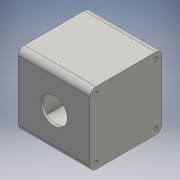
# Autodesk Inventor part: 60x60Motor
Saved by Autodesk Inventor 2016 (Build 200138000, 138)
## iProperties
Created: 2016-05-22
Part Number: 60x60Motor
Material: Generic
Document SubType Name: Modeling
Designer: Kurtis
Density: 1 g/cm^3
Appearance: Default
Author: Kurtis
Autodesk Inventor part; units mm, degrees
ref_plane "YZ Plane" through (0, 0, 0) normal (1, 0, 0) x (0, 1, 0)
ref_plane "XZ Plane" through (0, 0, 0) normal (0, 1, 0) x (-1, 0, 0)
ref_plane "XY Plane" through (0, 0, 0) normal (0, 0, 1) x (1, 0, 0)
sketch "Sketch1" plane through (0, 0, 0) normal (0, 0, 1) x (1, 0, 0)
  line L0 (-30, -30) -> (30, -30)
  line L1 (30, -30) -> (30, 30)
  line L2 (30, 30) -> (-30, 30)
  line L3 (-30, 30) -> (-30, -30)
  line L4 (-30, -30) -> (30, 30) construction
  line L5 (30, -30) -> (-30, 30) construction
  point P0 (0, 0)
  dimension "d0" = 60
  dimension "d1" = 60
  constraints: 12 end point, 2 midpoint, 2 parallel, 1 horizontal, 1 perpendicular
  measures "d0" distance of L2.end L1.end
  measures "d1" distance of L1.end L0.end
extrude "Main Block" add sketch "Sketch1" along normal blind 60
sketch "Sketch2" plane through (-30, 30, 0) normal (0, 1, 0) x (1, 0, 0)
  line L0 (0, -60) -> (60, -60) construction
  line L1 (0, 0) -> (60, 0) construction
  line L2 (60, -60) -> (0, 0) construction
  line L3 (51.25, -51.25) -> (8.75, -51.25)
  line L4 (8.75, -51.25) -> (8.75, -8.75)
  line L5 (8.75, -8.75) -> (51.25, -8.75)
  line L6 (51.25, -8.75) -> (51.25, -51.25)
  line L7 (51.25, -51.25) -> (8.75, -8.75) construction
  line L8 (8.75, -51.25) -> (51.25, -8.75) construction
  line L9 (30, -30) -> (30, -51.25) construction
  point P0 (30, 0)
  dimension "d4" = 42.5
  dimension "d5" = 42.5
  constraints: 16 end point, 4 midpoint, 2 parallel, 1 horizontal, 1 perpendicular
  measures "d4" distance of L4.end L5.end
  measures "d5" distance of L3.end L4.end
extrude "Motor Void" cut sketch "Sketch2" against normal blind 58
sketch "Sketch3" plane through (-30, 30, 0) normal (0, 1, 0) x (1, 0, 0)
  line L0 (30, 0) -> (30, -8.75) construction
  line L1 (8.75, -8.75) -> (51.25, -8.75) construction
  line L2 (38.25, 0.125) -> (21.75, 0.125)
  line L3 (21.75, 0.125) -> (21.75, -8.875)
  line L4 (21.75, -8.875) -> (38.25, -8.875)
  line L5 (38.25, -8.875) -> (38.25, 0.125)
  line L6 (38.25, 0.125) -> (21.75, -8.875) construction
  line L7 (21.75, 0.125) -> (38.25, -8.875) construction
  point P0 (30, -4.375)
  dimension "d30" = 16.5
  dimension "d31" = 9
  constraints: 14 end point, 4 midpoint, 2 parallel, 1 horizontal, 1 perpendicular
  measures "d30" distance of L4.end L3.end
  measures "d31" distance of L3.end L2.end
extrude "Cable Void" cut sketch "Sketch3" against normal blind 41
sketch "Sketch4" plane through (-30, -30, 0) normal (0, -1, 0) x (1, 0, 0)
  line L0 (0, 0) -> (0, 60) construction
  line L1 (60, 60) -> (0, 60) construction
  line L2 (0, 0) -> (60, 60) construction
  circle A0 centre (30, 30) radius 11
  point P0 (30, 0)
  dimension "d12" = 22
  constraints: 2 end point, 1 centre point, 1 midpoint
  measures "d12" diameter of A0
extrude "Raised Void" cut sketch "Sketch4" against normal blind 2
sketch "Sketch6" plane through (-30, -30, 0) normal (-1, 0, 0) x (0, 0, 1)
  line L0 (60, 0) -> (60, 60) construction
  line L1 (60, 60) -> (60, 55) construction
  line L2 (60, 55) -> (55, 55) construction
  line L3 (60, 0) -> (60, 5) construction
  line L4 (60, 5) -> (55, 5) construction
  line L5 (0, 0) -> (5, 0) construction
  line L6 (0, 0) -> (60, 0) construction
  line L7 (5, 0) -> (5, 5) construction
  line L8 (0, 60) -> (0, 0) construction
  line L9 (0, 60) -> (5, 60) construction
  line L10 (0, 60) -> (60, 60) construction
  line L11 (5, 60) -> (5, 55) construction
  circle A0 centre (55, 55) radius 1.5
  circle A1 centre (55, 5) radius 1.5
  circle A2 centre (5, 5) radius 1.5
  circle A3 centre (5, 55) radius 1.5
  point P0 (0, 30)
  dimension "d32" = 5
  dimension "d33" = 5
  dimension "d34" = 5
  dimension "d35" = 5
  dimension "d36" = 5
  dimension "d37" = 5
  dimension "d38" = 5
  dimension "d39" = 5
  dimension "d40" = 3
  dimension "d41" = 3
  dimension "d42" = 3
  dimension "d43" = 3
  constraints: 16 end point, 4 centre point, 4 coincident, 4 perpendicular, 4 point on line
  measures "d32" distance of L0.end L1.end
  measures "d33" distance of L1.end L2.end
  measures "d34" distance of L0.start L3.end
  measures "d35" distance of L3.end L4.end
  measures "d36" distance of L5.start L5.end
  measures "d37" distance of L5.end L7.end
  measures "d38" distance of L8.start L9.end
  measures "d39" distance of L9.end L11.end
  measures "d40" diameter of A0
  measures "d41" diameter of A1
  measures "d42" diameter of A2
  measures "d43" diameter of A3
extrude "Holes" cut sketch "Sketch6" against normal blind 60
fillet "Cleaning it up" radius 5 5 edges at (0, 30, 60) (0, -30, 60) (19.125, 30, 0) (-19.125, 30, 0) (0, -30, 0)
equation "\"d4\" = d5"
body "Solid1"
